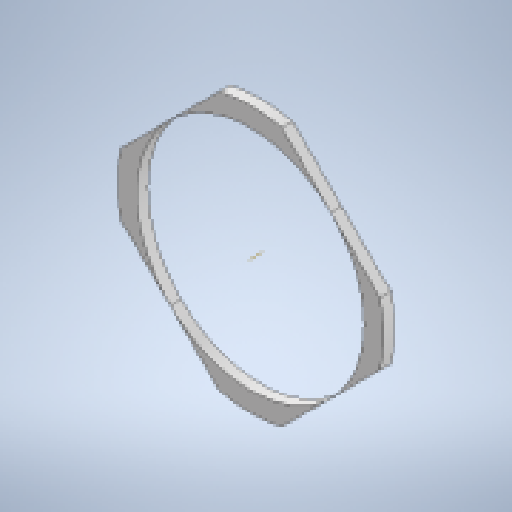
# Autodesk Inventor part: MainBaseCircle210
Saved by Autodesk Inventor 2025.1 (Build 291241000, 241)
## iProperties
Created: 2025-05-09
Part Number: MainBaseCircle210
Material: Generic
Document SubType Name: Modeling
Designer: User
Density: 1 g/cm^3
Appearance: Default
Author: User
Autodesk Inventor part; units mm, degrees
ref_plane "YZ Plane" through (0, 0, 0) normal (1, 0, 0) x (0, 1, 0)
ref_plane "XZ Plane" through (0, 0, 0) normal (0, 1, 0) x (-1, 0, 0)
ref_plane "XY Plane" through (0, 0, 0) normal (0, 0, 1) x (1, 0, 0)
sketch "Sketch1" plane through (0, 0, 0) normal (0, 0, 1) x (1, 0, 0)
  line L0 (20, 22.75) -> (-20, 22.75) projected
  line L1 (29, 73.2) -> (29, 63.2)
  line L2 (0, 22.75) -> (0, 135.7646)
  line L3 (29, 73.2) -> (0, 102.2)
  line L4 (29, 73.2) -> (70.0122, 73.2) construction
  line L5 (0, 102.2) -> (148.4924, -46.2924)
  line L6 (148.4924, -46.2924) -> (0, -194.7848)
  line L7 (0, -194.7848) -> (-148.4924, -46.2924)
  line L8 (-148.4924, -46.2924) -> (0, 102.2)
  line L9 (0, 102.2) -> (210, 102.2) construction
  line L10 (-74.2462, 27.9538) -> (74.2462, -120.5386)
  circle A0 centre (0, -46.2924) radius 122.9611
  circle A1 centre (0, -46.2924) radius 105
  point P0 (0, 0)
  point P1 (-74.2462, -120.5386)
  point P2 (-29, -165.7848)
  point P3 (29, -165.7848)
  point P4 (74.2462, 27.9538)
  point P5 (-29, 73.2)
  point P6 (119.4924, -75.2924)
  point P7 (119.4924, -17.2924)
  point P8 (-119.4924, -17.2924)
  point P9 (-119.4924, -75.2924)
  dimension "d0" = 135
  dimension "d1" = 210
  dimension "d2" = 45
  dimension "d3" = 210
  constraints: 20 end point, 4 midpoint, 2 equal length, 2 horizontal, 2 parallel, 2 vertical, 1 centre point, 1 coincident, 1 collinear, 1 perpendicular, 1 point on line, 5 other
  measures "d0" angle of L4 L3
  measures "d1" distance of L3.end L5.end
  measures "d2" angle of L5 L9
  measures "d3" distance of L5.end L6.end
extrude "Extrusion1" add sketch "Sketch1" along normal blind 10 contours A1 L8 A0 L2 | L2 A0 L5 A1 | L5 A0 L6 A1 | A1 L7 A0 L8 | L6 A0 L7 A1
body "Solid1"
